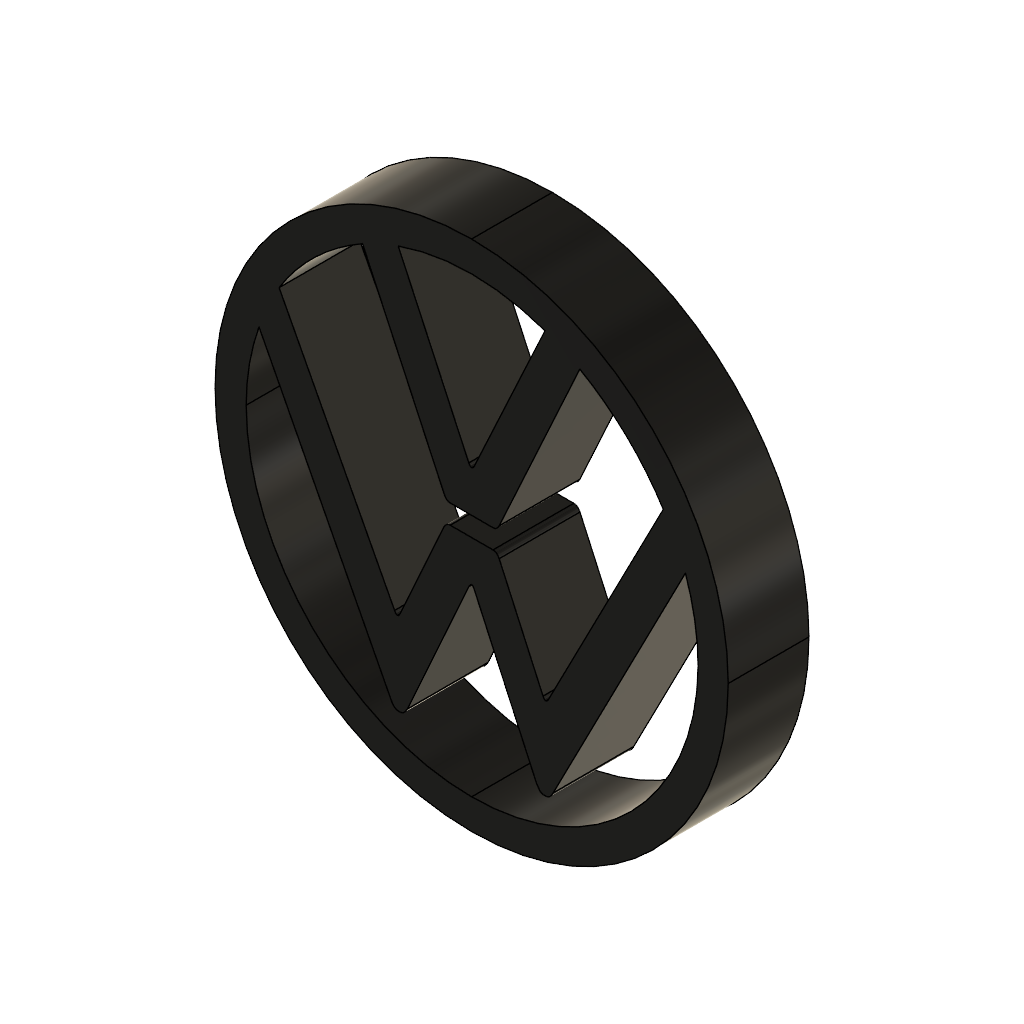
VolkswagenLogo (Autodesk Fusion 360 design; units mm, degrees)
part number: 2026-10-03-23-21-48-406
Autodesk Fusion 360 part; units mm, degrees
sketch "Sketch1" plane through (0, 0, 0) normal (0, 1, 0) x (1, 0, 0)
  spline S0 degree 3 poles (0, -3.15) (-1.7568, -3.15) (-3.175, -1.7318) (-3.175, 0.025) knots 0 0 0 0 1 1 1 1
  spline S1 degree 3 poles (-3.175, 0.025) (-3.175, 1.7818) (-1.7568, 3.2) (0, 3.2) knots 0 0 0 0 1 1 1 1
  spline S2 degree 3 poles (0, 3.2) (1.7568, 3.2) (3.175, 1.7818) (3.175, 0.025) knots 0 0 0 0 1 1 1 1
  spline S3 degree 3 poles (3.175, 0.025) (3.175, -1.7318) (1.7568, -3.15) (0, -3.15) knots 0 0 0 0 1 1 1 1
  spline S4 degree 3 poles (0, -2.7769) (0.3175, -2.7769) (0.6244, -2.7187) (0.9075, -2.6208) knots 0 0 0 0 1 1 1 1
  line L0 (0.9075, -2.6208) -> (0.0344, -0.7344)
  spline S5 degree 3 poles (0.0344, -0.7344) (0.0238, -0.7238) (0.0238, -0.7) (0, -0.7) knots 0 0 0 0 1 1 1 1
  spline S6 degree 3 poles (0, -0.7) (-0.0238, -0.7) (-0.0238, -0.7238) (-0.0344, -0.7344) knots 0 0 0 0 1 1 1 1
  line L1 (-0.0344, -0.7344) -> (-0.9075, -2.6208)
  line L2 (-1.3494, -2.425) -> (-0.3387, -0.2475)
  spline S7 degree 3 poles (-0.3387, -0.2475) (-0.3175, -0.2025) (-0.2937, -0.1893) (-0.2646, -0.1893) knots 0 0 0 0 1 1 1 1
  line L3 (-0.2646, -0.1893) -> (0.2646, -0.1893)
  spline S8 degree 3 poles (0.2646, -0.1893) (0.2963, -0.1893) (0.3175, -0.2025) (0.3413, -0.2475) knots 0 0 0 0 1 1 1 1
  line L4 (0.3413, -0.2475) -> (1.3388, -2.425)
  spline S9 degree 3 poles (1.3388, -2.425) (1.7568, -2.1869) (2.1167, -1.8456) (2.3707, -1.4381) knots 0 0 0 0 1 1 1 1
  line L5 (2.3707, -1.4381) -> (0.9525, 1.3056)
  spline S10 degree 3 poles (0.9525, 1.3056) (0.9419, 1.3294) (0.926, 1.34) (0.9181, 1.34) knots 0 0 0 0 1 1 1 1
  spline S11 degree 3 poles (0.9181, 1.34) (0.8969, 1.34) (0.8969, 1.3188) (0.8837, 1.3056) knots 0 0 0 0 1 1 1 1
  line L6 (0.8837, 1.3056) -> (0.3413, 0.1044)
  spline S12 degree 3 poles (0.3413, 0.1044) (0.3175, 0.0594) (0.2963, 0.0488) (0.2646, 0.0488) knots 0 0 0 0 1 1 1 1
  line L7 (0.2646, 0.0488) -> (-0.2646, 0.0488)
  spline S13 degree 3 poles (-0.2646, 0.0488) (-0.2937, 0.0488) (-0.3175, 0.0594) (-0.3413, 0.1044) knots 0 0 0 0 1 1 1 1
  line L8 (-0.3413, 0.1044) -> (-0.8837, 1.3056)
  spline S14 degree 3 poles (-0.8837, 1.3056) (-0.8969, 1.3188) (-0.8943, 1.34) (-0.9181, 1.34) knots 0 0 0 0 1 1 1 1
  spline S15 degree 3 poles (-0.9181, 1.34) (-0.9419, 1.34) (-0.9419, 1.3188) (-0.9525, 1.3056) knots 0 0 0 0 1 1 1 1
  line L9 (-0.9525, 1.3056) -> (-2.3812, -1.4381)
  spline S16 degree 3 poles (-2.3812, -1.4381) (-2.1325, -1.8456) (-1.7674, -2.1869) (-1.3494, -2.425) knots 0 0 0 0 1 1 1 1
  line L10 (-2.63, -0.8931) -> (-0.9975, 2.2819)
  spline S17 degree 3 poles (-0.9975, 2.2819) (-0.9763, 2.3269) (-0.9525, 2.3613) (-0.8943, 2.3613) knots 0 0 0 0 1 1 1 1
  spline S18 degree 3 poles (-0.8943, 2.3613) (-0.8387, 2.3613) (-0.8176, 2.3269) (-0.7937, 2.2819) knots 0 0 0 0 1 1 1 1
  line L11 (-0.7937, 2.2819) -> (-0.0344, 0.5912)
  spline S19 degree 3 poles (-0.0344, 0.5912) (-0.0238, 0.57) (-0.0106, 0.5542) (0, 0.5542) knots 0 0 0 0 1 1 1 1
  spline S20 degree 3 poles (0, 0.5542) (0.0238, 0.5542) (0.0238, 0.5806) (0.0344, 0.5912) knots 0 0 0 0 1 1 1 1
  line L12 (0.0344, 0.5912) -> (0.8043, 2.2819)
  spline S21 degree 3 poles (0.8043, 2.2819) (0.8281, 2.3269) (0.8493, 2.3613) (0.9075, 2.3613) knots 0 0 0 0 1 1 1 1
  spline S22 degree 3 poles (0.9075, 2.3613) (0.9631, 2.3613) (0.9869, 2.3269) (1.0081, 2.2819) knots 0 0 0 0 1 1 1 1
  line L13 (1.0081, 2.2819) -> (2.6458, -0.8931)
  spline S23 degree 3 poles (2.6458, -0.8931) (2.7437, -0.61) (2.8019, -0.3031) (2.8019, 0.025) knots 0 0 0 0 1 1 1 1
  spline S24 degree 3 poles (2.8019, 0.025) (2.7887, 1.5569) (1.5319, 2.8269) (0, 2.8269) knots 0 0 0 0 1 1 1 1
  spline S25 degree 3 poles (0, 2.8269) (-1.5319, 2.8269) (-2.7887, 1.5569) (-2.7887, 0.025) knots 0 0 0 0 1 1 1 1
  spline S26 degree 3 poles (-2.7887, 0.025) (-2.7887, -0.2925) (-2.7331, -0.5968) (-2.63, -0.8931) knots 0 0 0 0 1 1 1 1
  arc A0 (-0.9075, -2.6208) -> (0.9075, -2.6208) centre (0, -0.0609) ccw
  constraint coincident S4.start A0
  constraint coincident S4.end L0.start
  constraint coincident L1.end A0.start
extrude "Extrude2" add sketch "Sketch1" along normal blind 1
